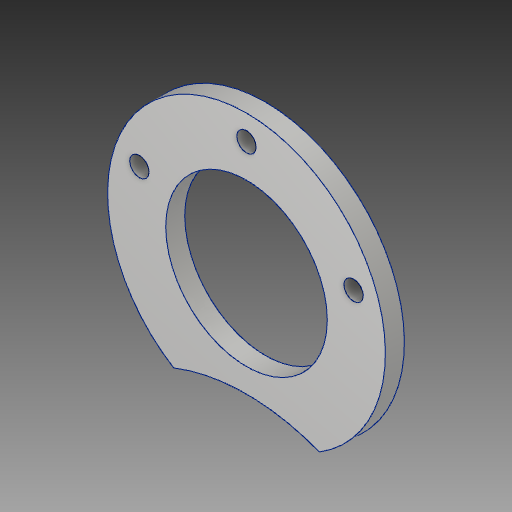
# Autodesk Inventor part: 円 42.5mm
Saved by Autodesk Inventor 2019 (Build 230136000, 136)
## iProperties
Created: 2020-09-27
Part Number: 円 42.5mm
Material: アルミニウム 6061
Document SubType Name: Modeling
Designer: Toshihito
Density: 2.7 g/cm^3
Appearance: アルミニウム - フラット
Mass: 33.5184 g
Surface Area: 70.1631 cm^2
Volume: 12.4142 cm^3
Author: Toshihito
Autodesk Inventor part; units mm, degrees
ref_plane "YZ Plane" through (0, 0, 0) normal (1, 0, 0) x (0, 1, 0)
ref_plane "XZ Plane" through (0, 0, 0) normal (0, 1, 0) x (-1, 0, 0)
ref_plane "XY Plane" through (0, 0, 0) normal (0, 0, 1) x (1, 0, 0)
sketch "スケッチ1" plane through (0, 0, 0) normal (0, 0, 1) x (1, 0, 0)
  circle A0 centre (0, 0) radius 21.25
  circle A1 centre (0, 0) radius 36.55
  line L0 (0, 0) -> (-28.1908, 10.2606) construction
  line L1 (0, 0) -> (28.1908, 10.2606) construction
  line L2 (-39.5959, 0) -> (43.1917, 0) construction
  line L3 (0, 0) -> (0, 30) construction
  circle A2 centre (-28.1908, 10.2606) radius 2.55
  circle A3 centre (0, 30) radius 2.55
  circle A4 centre (28.1908, 10.2606) radius 2.55
  dimension "d0" = 73.1
  dimension "d1" = 42.5
  dimension "d2" = 30
  dimension "d3" = 30
  dimension "d4" = 20
  dimension "d5" = 20
  dimension "d6" = 30
  dimension "d7" = 5.1
  dimension "d8" = 5.1
  dimension "d9" = 5.1
  constraints: 8 end point, 5 centre point, 5 coincident, 1 horizontal, 1 vertical
  measures "d0" diameter of A1
  measures "d1" diameter of A0
  measures "d2" distance of L0.start L0.end
  measures "d3" distance of L0.start L1.end
  measures "d4" angle of L2 L0
  measures "d5" angle of L2 L1
  measures "d6" distance of L0.start L3.end
  measures "d7" diameter of A2
  measures "d8" diameter of A3
  measures "d9" diameter of A4
extrude "押し出し1" add sketch "スケッチ1" along normal blind 5
sketch "スケッチ2" plane through (0, 0, 5) normal (0, 0, 1) x (1, 0, 0)
  line L0 (0, 0) -> (0, -80) construction
  circle A0 centre (0, -80) radius 52.5
  dimension "d12" = 80
  dimension "d16" = 105
  constraints: 2 end point, 1 centre point, 1 vertical
  measures "d12" distance of L0.start L0.end
  measures "d16" diameter of A0
extrude "押し出し2" cut sketch "スケッチ2" against normal blind 10
